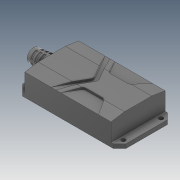
# Autodesk Inventor part: ESC
Saved by Autodesk Inventor 2020 (Build 240168000, 168)
## iProperties
Created: 2020-09-29
Part Number: ESC
Material: Generic
Document SubType Name: Modeling
Designer: DELL
Density: 1 g/cm^3
Appearance: Smooth - Black
Author: DELL
Autodesk Inventor part; units mm, degrees
ref_plane "YZ Plane" through (0, 0, 0) normal (1, 0, 0) x (0, 1, 0)
ref_plane "XZ Plane" through (0, 0, 0) normal (0, 1, 0) x (-1, 0, 0)
ref_plane "XY Plane" through (0, 0, 0) normal (0, 0, 1) x (1, 0, 0)
sketch "Sketch1" plane through (0, 0, 0) normal (0, 1, 0) x (-1, 0, 0)
  line L0 (-24.7, -12.9) -> (24.7, -12.9)
  line L1 (24.7, -12.9) -> (24.7, 12.9)
  line L2 (24.7, 12.9) -> (-24.7, 12.9)
  line L3 (-24.7, 12.9) -> (-24.7, -12.9)
  line L4 (-24.7, -12.9) -> (24.7, 12.9) construction
  line L5 (24.7, -12.9) -> (-24.7, 12.9) construction
  point P0 (0, 0)
  dimension "d0" = 49.4
  dimension "d1" = 25.8
  constraints: 12 end point, 2 midpoint, 2 parallel, 1 horizontal, 1 perpendicular
  measures "d0" distance between parallel lines of L3 L1
  measures "d1" distance of L0.end L1.end
extrude "Extrusion1" add sketch "Sketch1" along normal blind 2
chamfer "Chamfer1" distance 3 angle 45 4 edges at (24.7, 1, 12.9) (24.7, 1, -12.9) (-24.7, 1, 12.9) (-24.7, 1, -12.9)
sketch "Sketch2" plane through (0, 2, 0) normal (0, 1, 0) x (1, 0, 0)
  circle A0 centre (22.6, -9) radius 1
  circle A1 centre (22.6, 9) radius 1
  circle A2 centre (-22.6, -9) radius 1
  circle A3 centre (-22.6, 9) radius 1
  line L0 (24.7, -9.9) -> (24.7, 9.9) construction
  line L1 (24.7, 0) -> (-24.7, 0) construction
  line L2 (-24.7, 9.9) -> (-24.7, -9.9) construction
  line L3 (-21.7, -12.9) -> (21.7, -12.9) construction
  line L4 (0, -12.9) -> (0, 13.4418) construction
  point P0 (0, 0)
  dimension "d7" = 2
  dimension "d8" = 45.2
  dimension "d9" = 18
  constraints: 4 centre point, 4 end point, 3 equal radius, 3 midpoint, 2 horizontal alignment, 2 symmetric about line, 2 vertical alignment, 1 vertical
  measures "d7" diameter of A0
  measures "d8" distance of A2.centre A0.centre
  measures "d9" distance of A1.centre A0.centre
extrude "Extrusion2" cut sketch "Sketch2" against normal up to surface (2 mm away)
ref_plane "Work Plane1" through (0, 0, 9.9) normal (1, 0, 0) x (0, 0, -1)
sketch "Sketch3" plane through (0, 0, 9.9) normal (1, 0, 0) x (0, 0, -1)
  line L0 (22.8, 2) -> (19.8, 2) projected
  line L1 (22.8, 2) -> (22.8, 10.5)
  line L2 (22.8, 10.5) -> (16.4, 11.5)
  line L3 (16.4, 11.5) -> (3.4, 11.5)
  line L4 (3.4, 11.5) -> (-3, 10.5)
  line L5 (-3, 10.5) -> (-3, 2)
  line L6 (-0.1, 2) -> (1.9, 2) projected
  line L7 (22.8, 2) -> (-3, 2)
  line L8 (22.8, 0) -> (22.8, 2) projected
  line L9 (-3, 2) -> (-3, 0) projected
  line L10 (0, 0) -> (19.8, 0) projected
  line L11 (9.9, 0) -> (9.9, 11.5) construction
  line L12 (-3, 0) -> (0, 0) construction
  dimension "d12" = 11.5
  dimension "d13" = 13
  dimension "d14" = 10.5
  constraints: 14 end point, 3 perpendicular, 2 collinear, 2 point on line, 1 midpoint, 1 parallel, 1 vertical, 1 other
  measures "d12" distance between parallel lines of L10 L3
  measures "d13" distance of L2.end L3.end
  measures "d14" distance from line of L4.end L12
extrude "Extrusion3" add sketch "Sketch3" along normal mid plane 41.2
sketch "Sketch4" plane through (-20.6, 11.5, 6.5) normal (0, 1, 0) x (1, 0, 0)
  line L0 (42.3, 19.4) -> (-1.1, 19.4) projected
  line L1 (12.5522, 19.4) -> (20, 6.5)
  line L2 (20, 6.5) -> (12.5522, -6.4)
  line L3 (-1.1, -6.4) -> (42.3, -6.4) projected
  line L4 (14.8616, 19.4) -> (22.3094, 6.5)
  line L5 (22.3094, 6.5) -> (14.8616, -6.4)
  line L6 (12.5522, -6.4) -> (14.8616, -6.4)
  line L7 (12.5522, 19.4) -> (14.8616, 19.4)
  line L8 (20.6, 6.5) -> (-4.1, 6.5) construction
  line L9 (-4.1, 16.4) -> (-4.1, -3.4) construction
  line L10 (0, 0) -> (0, 13) construction
  line L11 (17.171, 19.4) -> (21.2124, 12.4)
  line L12 (21.2124, 12.4) -> (31.1295, 12.4)
  line L13 (31.1295, 12.4) -> (35.171, 19.4)
  line L14 (26.171, 12.4) -> (26.171, 19.4) construction
  line L15 (17.171, -6.4) -> (21.2124, 0.6)
  line L16 (21.2124, 0.6) -> (31.1295, 0.6)
  line L17 (31.1295, 0.6) -> (35.171, -6.4)
  point P0 (35.171, -6.4)
  dimension "d17" = 2
  dimension "d18" = 2
  dimension "d19" = 120
  dimension "d20" = 20
  dimension "d21" = 2
  dimension "d22" = 7
  dimension "d23" = 18
  constraints: 28 end point, 8 point on line, 4 symmetric about line, 3 horizontal, 3 parallel, 2 midpoint, 1 perpendicular, 1 vertical alignment, 1 other
  measures "d17" distance between parallel lines of L4 L1
  measures "d18" distance between parallel lines of L5 L2
  measures "d19" angle of L2 L1
  measures "d20" distance from line of L10 L1.end
  measures "d21" distance between parallel lines of L4 L11
  measures "d22" distance between parallel lines of L0 L12
  measures "d23" distance of L13.end L11.start
extrude "Extrusion4" cut sketch "Sketch4" against normal blind 1
fillet "Fillet1" radius 2 6 edges at (1.7094, 11, 0) (-0.6, 11, 0) (0.6124, 11, 5.9) (10.5295, 11, 5.9) (10.5295, 11, -5.9) (0.6124, 11, -5.9)
sketch "Sketch6" plane through (-20.6, 0, 9.9) normal (-1, 0, 0) x (0, 0, 1)
  circle A0 centre (-9.9, 6.75) radius 4
  line L0 (-16.4, 11.5) -> (-3.4, 11.5) construction
  line L1 (-9.9, 11.5) -> (-9.9, 0) construction
  line L2 (-22.8, 2) -> (-22.8, 10.5) construction
  line L3 (-22.8, 6.75) -> (3, 6.75) construction
  line L4 (3, 10.5) -> (3, 2) construction
  point P0 (-9.9, 6.75)
  dimension "d27" = 8
  dimension "d28" = 4.75
  constraints: 4 end point, 2 midpoint, 2 point on line, 1 centre point, 1 coincident, 1 horizontal, 1 perpendicular
  measures "d27" diameter of A0
  measures "d28" distance between parallel lines of L0 L3
ref_plane "Work Plane2" through (-29.4, 0, 9.9) normal (-1, 0, 0) x (0, 0, 1)
sketch "Sketch7" plane through (-29.4, 0, 9.9) normal (-1, 0, 0) x (0, 0, 1)
  circle A0 centre (-9.9, 6.75) radius 3
  point P0 (-9.9, 0)
  dimension "d30" = 6
  constraints: 1 centre point, 1 coincident
  measures "d30" diameter of A0
loft "Loft1" add profiles "Sketch6", "Sketch7"
ref_plane "Work Plane3" through (-21.6, 0, 9.9) normal (-1, 0, 0) x (0, 0, 1)
sketch "Sketch8" plane through (-21.6, 0, 9.9) normal (-1, 0, 0) x (0, 0, 1)
  circle A0 centre (-9.9, 6.75) radius 4 projected
  circle A1 centre (-9.9, 6.75) radius 3.8847
  circle A2 centre (-9.9, 6.75) radius 3.388
  line L0 (-9.4, 2.75) -> (-10.4, 2.75)
  line L1 (-10.4, 2.75) -> (-10.4, 10.75)
  line L2 (-10.4, 10.75) -> (-9.4, 10.75)
  line L3 (-9.4, 10.75) -> (-9.4, 2.75)
  line L4 (-9.4, 2.75) -> (-10.4, 10.75) construction
  line L5 (-10.4, 2.75) -> (-9.4, 10.75) construction
  line L6 (-5.9, 7.25) -> (-13.9, 7.25)
  line L7 (-13.9, 7.25) -> (-13.9, 6.25)
  line L8 (-13.9, 6.25) -> (-5.9, 6.25)
  line L9 (-5.9, 6.25) -> (-5.9, 7.25)
  line L10 (-5.9, 7.25) -> (-13.9, 6.25) construction
  line L11 (-13.9, 7.25) -> (-5.9, 6.25) construction
  point P0 (-9.9, 0)
  point P1 (-13.2509, 6.25)
  point P2 (-13.7524, 6.25)
  point P3 (-10.4, 2.8976)
  point P4 (-10.4, 3.3991)
  point P5 (-13.7524, 7.25)
  point P6 (-13.2509, 7.25)
  point P7 (-10.4, 10.1009)
  point P8 (-10.4, 10.6024)
  dimension "d36" = 6.776
  dimension "d37" = 1
  dimension "d38" = 1
  constraints: 24 end point, 4 midpoint, 4 parallel, 2 centre point, 2 coincident, 2 horizontal, 2 perpendicular, 2 tangent
  measures "d36" diameter of A2
  measures "d37" distance of L1.end L2.end
  measures "d38" distance of L6.end L7.end
extrude "Extrusion5" cut sketch "Sketch8" along normal blind 1 contours L1 A2 L6 A1 | A1 L8 A2 L1
ref_plane "Work Plane4" through (-22.6, 0, 9.9) normal (-1, 0, 0) x (0, 0, 1)
sketch "Sketch9" plane through (-22.6, 0, 9.9) normal (-1, 0, 0) x (0, 0, 1)
  circle A0 centre (-9.9, 6.75) radius 4 projected
  circle A1 centre (-9.9, 6.75) radius 4
  circle A2 centre (-9.9, 6.75) radius 3.2885
  line L0 (-9.4, 2.75) -> (-10.4, 2.75)
  line L1 (-10.4, 2.75) -> (-10.4, 10.75)
  line L2 (-10.4, 10.75) -> (-9.4, 10.75)
  line L3 (-9.4, 10.75) -> (-9.4, 2.75)
  line L4 (-9.4, 2.75) -> (-10.4, 10.75) construction
  line L5 (-10.4, 2.75) -> (-9.4, 10.75) construction
  line L6 (-5.9, 7.25) -> (-13.9, 7.25)
  line L7 (-13.9, 7.25) -> (-13.9, 6.25)
  line L8 (-13.9, 6.25) -> (-5.9, 6.25)
  line L9 (-5.9, 6.25) -> (-5.9, 7.25)
  line L10 (-5.9, 7.25) -> (-13.9, 6.25) construction
  line L11 (-13.9, 7.25) -> (-5.9, 6.25) construction
  point P0 (-9.9, 0)
  point P1 (-5.9314, 6.25)
  point P2 (-6.6497, 6.25)
  point P3 (-9.4, 3.4997)
  point P4 (-9.4, 2.7814)
  point P5 (-6.6497, 7.25)
  point P6 (-5.9314, 7.25)
  point P7 (-9.4, 10.7186)
  point P8 (-9.4, 10.0003)
  dimension "d42" = 6.577
  dimension "d43" = 1
  dimension "d44" = 1
  dimension "d45" = 8
  constraints: 24 end point, 4 midpoint, 4 parallel, 2 centre point, 2 coincident, 2 horizontal, 2 perpendicular, 2 tangent
  measures "d42" diameter of A2
  measures "d43" distance of L1.end L2.end
  measures "d44" distance of L6.end L7.end
  measures "d45" diameter of A1
extrude "Extrusion6" cut sketch "Sketch9" along normal blind 1 contours L6 A2 L3 A0 | A0 L3 A2 L8
ref_plane "Work Plane5" through (-23.6, 0, 9.9) normal (-1, 0, 0) x (0, 0, 1)
sketch "Sketch10" plane through (-23.6, 0, 9.9) normal (-1, 0, 0) x (0, 0, 1)
  circle A0 centre (-9.9, 6.75) radius 4 projected
  circle A1 centre (-9.9, 6.75) radius 3.169
  circle A2 centre (-9.9, 6.75) radius 3.9804
  line L0 (-9.4, 2.75) -> (-10.4, 2.75)
  line L1 (-10.4, 2.75) -> (-10.4, 10.75)
  line L2 (-10.4, 10.75) -> (-9.4, 10.75)
  line L3 (-9.4, 10.75) -> (-9.4, 2.75)
  line L4 (-9.4, 2.75) -> (-10.4, 10.75) construction
  line L5 (-10.4, 2.75) -> (-9.4, 10.75) construction
  line L6 (-5.9, 7.25) -> (-13.9, 7.25)
  line L7 (-13.9, 7.25) -> (-13.9, 6.25)
  line L8 (-13.9, 6.25) -> (-5.9, 6.25)
  line L9 (-5.9, 6.25) -> (-5.9, 7.25)
  line L10 (-5.9, 7.25) -> (-13.9, 6.25) construction
  line L11 (-13.9, 7.25) -> (-5.9, 6.25) construction
  point P0 (-9.9, 0)
  point P1 (-13.0293, 6.25)
  point P2 (-13.8489, 6.25)
  point P3 (-10.4, 2.8011)
  point P4 (-10.4, 3.6207)
  point P5 (-13.8489, 7.25)
  point P6 (-13.0293, 7.25)
  point P7 (-10.4, 9.8793)
  point P8 (-10.4, 10.6989)
  dimension "d49" = 6.338
  dimension "d50" = 1
  dimension "d51" = 1
  constraints: 24 end point, 4 midpoint, 4 parallel, 2 centre point, 2 coincident, 2 horizontal, 2 perpendicular, 2 tangent
  measures "d49" diameter of A1
  measures "d50" distance of L1.end L2.end
  measures "d51" distance of L6.end L7.end
extrude "Extrusion7" cut sketch "Sketch10" along normal blind 1 contours L1 A2 L6 A0 | L1 A1 L6 A2 | A0 L8 A2 L1 | A2 L8 A1 L1
ref_plane "Work Plane6" through (-24.6, 0, 9.9) normal (-1, 0, 0) x (0, 0, 1)
sketch "Sketch11" plane through (-24.6, 0, 9.9) normal (-1, 0, 0) x (0, 0, 1)
  circle A0 centre (-9.9, 6.75) radius 4 projected
  circle A1 centre (-9.9, 6.75) radius 3.924
  circle A2 centre (-9.9, 6.75) radius 3.0305
  line L0 (-9.4, 2.75) -> (-10.4, 2.75)
  line L1 (-10.4, 2.75) -> (-10.4, 10.75)
  line L2 (-10.4, 10.75) -> (-9.4, 10.75)
  line L3 (-9.4, 10.75) -> (-9.4, 2.75)
  line L4 (-9.4, 2.75) -> (-10.4, 10.75) construction
  line L5 (-10.4, 2.75) -> (-9.4, 10.75) construction
  line L6 (-5.9, 7.25) -> (-13.9, 7.25)
  line L7 (-13.9, 7.25) -> (-13.9, 6.25)
  line L8 (-13.9, 6.25) -> (-5.9, 6.25)
  line L9 (-5.9, 6.25) -> (-5.9, 7.25)
  line L10 (-5.9, 7.25) -> (-13.9, 6.25) construction
  line L11 (-13.9, 7.25) -> (-5.9, 6.25) construction
  point P0 (-9.9, 0)
  point P1 (-6.008, 6.25)
  point P2 (-6.911, 6.25)
  point P3 (-9.4, 3.761)
  point P4 (-9.4, 2.858)
  point P5 (-6.911, 7.25)
  point P6 (-6.008, 7.25)
  point P7 (-9.4, 10.642)
  point P8 (-9.4, 9.739)
  dimension "d55" = 6.061
  dimension "d56" = 1
  dimension "d57" = 1
  constraints: 24 end point, 4 midpoint, 4 parallel, 2 centre point, 2 coincident, 2 horizontal, 2 perpendicular, 2 tangent
  measures "d55" diameter of A2
  measures "d56" distance of L1.end L2.end
  measures "d57" distance of L6.end L7.end
extrude "Extrusion8" cut sketch "Sketch11" along normal blind 1 contours L6 A2 L3 A1 | A1 L3 A2 L8
ref_plane "Work Plane7" through (-25.6, 0, 9.9) normal (-1, 0, 0) x (0, 0, 1)
sketch "Sketch12" plane through (-25.6, 0, 9.9) normal (-1, 0, 0) x (0, 0, 1)
  circle A0 centre (-9.9, 6.75) radius 4 projected
  circle A1 centre (-9.9, 6.75) radius 4.1817
  circle A2 centre (-9.9, 6.75) radius 2.9355
  line L0 (-10.4, 2.5683) -> (-9.4, 2.5683)
  line L1 (-9.4, 2.5683) -> (-9.4, 10.9317)
  line L2 (-9.4, 10.9317) -> (-10.4, 10.9317)
  line L3 (-10.4, 10.9317) -> (-10.4, 2.5683)
  line L4 (-10.4, 2.5683) -> (-9.4, 10.9317) construction
  line L5 (-9.4, 2.5683) -> (-10.4, 10.9317) construction
  line L6 (-5.7183, 7.25) -> (-14.0817, 7.25)
  line L7 (-14.0817, 7.25) -> (-14.0817, 6.25)
  line L8 (-14.0817, 6.25) -> (-5.7183, 6.25)
  line L9 (-5.7183, 6.25) -> (-5.7183, 7.25)
  line L10 (-5.7183, 7.25) -> (-14.0817, 6.25) construction
  line L11 (-14.0817, 7.25) -> (-5.7183, 6.25) construction
  point P0 (-9.9, 0)
  point P1 (-12.7926, 6.25)
  point P2 (-13.8686, 6.25)
  point P3 (-10.4, 2.7814)
  point P4 (-10.4, 3.8574)
  point P5 (-13.8686, 7.25)
  point P6 (-12.7926, 7.25)
  point P7 (-10.4, 9.6426)
  point P8 (-10.4, 10.7186)
  dimension "d61" = 5.871
  dimension "d62" = 1
  dimension "d63" = 1
  constraints: 24 end point, 4 midpoint, 4 parallel, 2 centre point, 2 coincident, 2 horizontal, 2 perpendicular, 2 tangent
  measures "d61" diameter of A2
  measures "d62" distance of L1.end L2.end
  measures "d63" distance of L6.end L7.end
extrude "Extrusion9" cut sketch "Sketch12" along normal blind 1 contours L3 A2 L6 A0 | A0 L8 A2 L3
ref_plane "Work Plane8" through (-26.6, 0, 9.9) normal (-1, 0, 0) x (0, 0, 1)
sketch "Sketch13" plane through (-26.6, 0, 9.9) normal (-1, 0, 0) x (0, 0, 1)
  circle A0 centre (-9.9, 6.75) radius 4 projected
  circle A1 centre (-9.9, 6.75) radius 3.6503
  circle A2 centre (-9.9, 6.75) radius 2.774
  line L0 (-9.4, 3.0997) -> (-10.4, 3.0997)
  line L1 (-10.4, 3.0997) -> (-10.4, 10.4003)
  line L2 (-10.4, 10.4003) -> (-9.4, 10.4003)
  line L3 (-9.4, 10.4003) -> (-9.4, 3.0997)
  line L4 (-9.4, 3.0997) -> (-10.4, 10.4003) construction
  line L5 (-10.4, 3.0997) -> (-9.4, 10.4003) construction
  line L6 (-6.2497, 7.25) -> (-13.5503, 7.25)
  line L7 (-13.5503, 7.25) -> (-13.5503, 6.25)
  line L8 (-13.5503, 6.25) -> (-6.2497, 6.25)
  line L9 (-6.2497, 6.25) -> (-6.2497, 7.25)
  line L10 (-6.2497, 7.25) -> (-13.5503, 6.25) construction
  line L11 (-13.5503, 7.25) -> (-6.2497, 6.25) construction
  point P0 (-9.9, 0)
  point P1 (-6.2841, 6.25)
  point P2 (-7.1714, 6.25)
  point P3 (-9.4, 4.0214)
  point P4 (-9.4, 3.1341)
  point P5 (-7.1714, 7.25)
  point P6 (-6.2841, 7.25)
  point P7 (-9.4, 10.3659)
  point P8 (-9.4, 9.4786)
  dimension "d67" = 5.548
  dimension "d68" = 1
  dimension "d69" = 1
  constraints: 24 end point, 4 midpoint, 4 parallel, 2 centre point, 2 coincident, 2 horizontal, 2 perpendicular, 2 tangent
  measures "d67" diameter of A2
  measures "d68" distance of L1.end L2.end
  measures "d69" distance of L6.end L7.end
extrude "Extrusion10" cut sketch "Sketch13" along normal blind 1 contours L6 A2 L3 A1 | A1 L3 A2 L8
body "Solid1"
